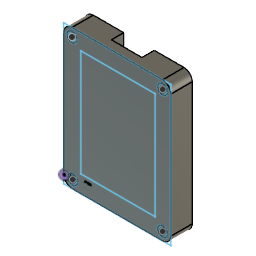
BluePrint (Autodesk Fusion 360 design; units mm, degrees)
part number: 2025-12-14-14-41-25-400
part number: 2025-12-14-14-47-09-582
Autodesk Fusion 360 part; units mm, degrees
sketch "Sketch1" plane through (0, 0, 0) normal (0, 1, 0) x (1, 0, 0) in component "JP's Hackpad"
  line L0 (10, -70) -> (55, -70)
  line L1 (55, -70) -> (55, -5.4)
  line L2 (55, -5.4) -> (10, -5.4)
  line L3 (10, -5.4) -> (10, -70)
  line L4 (-0.5, -79.5) -> (64.5, -79.5)
  line L5 (64.5, -79.5) -> (64.5, 5.1)
  line L6 (64.5, 5.1) -> (-0.5, 5.1)
  line L7 (-0.5, 5.1) -> (-0.5, -79.5)
  circle A0 centre (5, 0.1) radius 1.7
  circle A1 centre (4.5, -74.5) radius 1.7
  circle A2 centre (59.5, -74.5) radius 1.7
  circle A3 centre (59.5, 0.1) radius 1.7
  circle A4 centre (4.5, -74.5) radius 3
  circle A5 centre (59.5, -74.5) radius 3
  circle A6 centre (59.5, 0.1) radius 3
  circle A7 centre (5, 0.1) radius 3
  dimension "d1" = 64.6
  dimension "d2" = 45
  dimension "d3" = 84.6
  dimension "d4" = 65
  dimension "d5" = 9.5
  dimension "d6" = 9.5
  dimension "d7" = 3.4
  dimension "d8" = 5
  dimension "d9" = 5
  dimension "d10" = 3.4
  dimension "d11" = 5
  dimension "d12" = 5
  dimension "d13" = 3.4
  dimension "d14" = 5
  dimension "d15" = 5
  dimension "d16" = 3.4
  dimension "d17" = 5
  dimension "d18" = 5
  dimension "d19" = 6
  dimension "d20" = 6
  dimension "d21" = 6
  dimension "d22" = 6
  constraint horizontal L0
  constraint vertical L1
  constraint horizontal L2
  constraint vertical L3
  constraint horizontal L4
  constraint vertical L5
  constraint horizontal L6
  constraint vertical L7
  constraint coincident A1.centre A4.centre
  constraint coincident A2.centre A5.centre
  constraint coincident A3.centre A6.centre
  constraint coincident A0.centre A7.centre
  measures "d1" distance of L0.start L2.end
  measures "d2" distance of L0.start L0.end
  measures "d3" distance of L4.start L6.end
  measures "d4" distance of L4.start L4.end
  measures "d5" distance of L0 L4
  measures "d6" distance of L1 L5
  measures "d7" diameter of A0
  measures "d8" vertical distance of L6.end A0.centre
  measures "d9" horizontal distance of origin A0.centre
  measures "d10" diameter of A1
  measures "d11" distance of L4 A1.centre
  measures "d12" distance of L7 A1.centre
  measures "d13" diameter of A2
  measures "d14" distance of L4 A2.centre
  measures "d15" distance of L5 A2.centre
  measures "d16" diameter of A3
  measures "d17" distance of L5 A3.centre
  measures "d18" distance of L6 A3.centre
  measures "d19" diameter of A4
  measures "d20" diameter of A5
  measures "d21" diameter of A6
  measures "d22" diameter of A7
extrude "Extrude1" add sketch "Sketch1" along normal blind 9.9 from surface at 3.1 contours A4 | A5 | A6 | A7 makes body 1 at (7.3191, 9.7, 75.5261) makes body 2 at (7.9963, 9.7, 0.0495) makes body 3 at (62.0599, 9.7, 72.9357) makes body 4 at (62.4963, 9.7, 0.0495) in component "JP's Hackpad"
extrude "Extrude2" add sketch "Sketch1" along normal blind 13 contours L4 L5 L6 L7 bodies 1 2 3 4 in component "JP's Hackpad"
extrude "Extrude3" add sketch "Sketch1" along normal blind 3 contours L0 L1 L2 L3 bodies 1 in component "JP's Hackpad"
sketch "Sketch2" plane through (0, 13, 0) normal (0, 1, 0) x (-1, 0, 0) in component "JP's Hackpad"
  circle A0 centre (-4.5, 74.5) radius 1.7
  circle A1 centre (-59.5, -0.1) radius 1.7
  line L0 (-10, 70) -> (-10, 5.4)
  line L1 (-10, 5.4) -> (-55, 5.4)
  line L2 (-55, 5.4) -> (-55, 70)
  line L3 (-55, 70) -> (-10, 70)
  line L4 (0.5, -5.1) -> (0.5, 79.5)
  line L5 (0.5, 79.5) -> (-64.5, 79.5)
  line L6 (-64.5, 79.5) -> (-64.5, -5.1)
  line L7 (-64.5, -5.1) -> (0.5, -5.1)
  circle A2 centre (-5, -0.1) radius 1.7
  circle A3 centre (-59.5, 74.5) radius 1.7
  line L8 (-41.45, 79.5) -> (-22.95, 79.5)
  line L9 (-22.95, 79.5) -> (-22.95, 70)
  line L10 (-22.95, 70) -> (-41.45, 70)
  line L11 (-41.45, 70) -> (-41.45, 79.5)
  line L12 (-64.5, 79.5) -> (-64.5, -5.1)
  dimension "d30" = 18.5
  dimension "d31" = 23.05
  constraint horizontal L8
  constraint vertical L9
  constraint horizontal L10
  constraint vertical L11
  constraint coincident L3 L9.end
  constraint coincident L5 L8.start
  measures "d30" distance of L8.start L8.end
  measures "d31" distance of L11 L12
extrude "Extrude4" cut sketch "Sketch2" against normal blind 7.5 contours L3 L5 L8 L9 L10 L11 bodies 1 in component "JP's Hackpad"
fillet "Fillet1" radius 5 4 edges at (64.5, 6.5, 79.5) (-0.5, 6.5, 79.5) (64.5, 6.5, -5.1) (-0.5, 6.5, -5.1) on bodies 1 in component "JP's Hackpad"
sketch "Sketch1 (2)" plane through (0, 0, 0) normal (0, 1, 0) x (1, 0, 0)
  line L0 (12, 0) -> (35, 0) construction
  line L1 (35, 0) -> (35, -3) construction
  line L2 (35, -3) -> (12, -3) construction
  line L3 (12, -3) -> (12, 0) construction
  dimension "d36" = 1
  dimension "d37" = 0
  text T0 "JP 001" font "Arial" height 1 align left top in box 23 x 3 at (12, 0) x (1, 0) y (0, -1) spacing 1 kerned
extrude "Extrude5" cut sketch "Sketch1 (2)" along normal blind 0.2 text T0 bodies 1 in component "JP's Hackpad"
component "JP's Hackpad" placed x (1, 0, 0) y (0, 1, 0) z (0, 0, 1) at (0, 0, 0)
equation "d37 = 'JP 001'"
